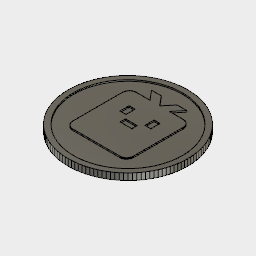
Tomato Coaster (Autodesk Fusion 360 design; units mm, degrees)
Autodesk Fusion 360 part; units mm, degrees
sketch "tomato" plane through (0, 0, 0) normal (0, 0, 1) x (1, 0, 0)
  line L0 (18.3031, 41.1095) -> (16.1266, 42.0111)
  line L1 (-21.8898, 21.7819) -> (-21.7279, 21.9929)
  line L2 (-22.0404, 21.5628) -> (-21.8898, 21.7819)
  line L3 (40.0953, 20.4296) -> (38.9711, 22.5)
  line L4 (22.853, 19.0619) -> (22.86, 18.796)
  line L5 (38.9711, 22.5) -> (37.7402, 24.5087)
  line L6 (-18.5747, 23.8134) -> (-18.311, 23.8482)
  line L7 (-30.1109, -33.4415) -> (-28.3194, -34.9716)
  line L8 (7.112, 12.4968) -> (7.112, 5.588)
  line L9 (-4.4196, 2.54) -> (-4.4196, -1.524)
  line L10 (-26.4503, -36.4058) -> (-24.5087, -37.7402)
  line L11 (44.7535, -4.7038) -> (44.9383, -2.3551)
  line L12 (28.3194, 34.9716) -> (26.4503, 36.4058)
  line L13 (-21.5552, 22.1952) -> (-21.3721, 22.3881)
  line L14 (42.0111, -16.1266) -> (42.7975, -13.9058)
  line L15 (-19.6005, 23.5386) -> (-19.3498, 23.6273)
  line L16 (-22.4208, -20.8622) -> (-22.5226, -20.6165)
  line L17 (-19.3498, 23.6273) -> (-19.0948, 23.7029)
  line L18 (-21.7279, 21.9929) -> (-21.5552, 22.1952)
  line L19 (20.0863, -23.3223) -> (19.8462, -23.4368)
  line L20 (-22.853, 19.0619) -> (-22.8322, 19.327)
  line L21 (-22.8322, 19.327) -> (-22.7975, 19.5907)
  line L22 (-30.1109, 33.4415) -> (-31.8198, 31.8198)
  line L23 (20.32, -23.1954) -> (20.0863, -23.3223)
  line L24 (19.8462, -23.4368) -> (19.6005, -23.5386)
  line L25 (19.6005, -23.5386) -> (19.3498, -23.6273)
  line L26 (11.5824, 12.4968) -> (7.112, 12.4968)
  line L27 (17.78, -23.876) -> (-17.78, -23.876)
  line L28 (22.5, 38.9711) -> (20.4296, 40.0953)
  line L29 (-34.9716, 28.3194) -> (-36.4058, 26.4503)
  line L30 (33.4415, -30.1109) -> (34.9716, -28.3194)
  line L31 (7.112, 5.588) -> (11.5824, 5.588)
  line L32 (44.446, -7.0396) -> (44.7535, -4.7038)
  line L33 (20.9769, -22.7439) -> (20.7659, -22.9058)
  line L34 (22.5, -38.9711) -> (24.5087, -37.7402)
  line L35 (-21.1792, -22.5712) -> (-21.3721, -22.3881)
  line L36 (-20.9769, -22.7439) -> (-21.1792, -22.5712)
  line L37 (19.0948, 23.7029) -> (19.3498, 23.6273)
  line L38 (-37.7402, -24.5087) -> (-36.4058, -26.4503)
  line L39 (31.8198, -31.8198) -> (33.4415, -30.1109)
  line L40 (36.4058, -26.4503) -> (37.7402, -24.5087)
  line L41 (-20.9769, 22.7439) -> (-20.7659, 22.9058)
  line L42 (37.7402, -24.5087) -> (38.9711, -22.5)
  line L43 (-20.32, 23.1954) -> (-20.0863, 23.3223)
  line L44 (-20.0863, 23.3223) -> (-19.8462, 23.4368)
  line L45 (-24.5087, -37.7402) -> (-22.5, -38.9711)
  line L46 (-21.1792, 22.5712) -> (-20.9769, 22.7439)
  line L47 (-20.5468, 23.0564) -> (-20.32, 23.1954)
  line L48 (-20.7659, 22.9058) -> (-20.5468, 23.0564)
  line L49 (-21.3721, 22.3881) -> (-21.1792, 22.5712)
  line L50 (44.0166, -9.356) -> (44.446, -7.0396)
  line L51 (-11.6469, -43.4667) -> (-9.356, -44.0166)
  line L52 (-13.9058, -42.7975) -> (-11.6469, -43.4667)
  line L53 (-16.1266, -42.0111) -> (-13.9058, -42.7975)
  line L54 (-18.3031, -41.1095) -> (-16.1266, -42.0111)
  line L55 (-20.4296, -40.0953) -> (-18.3031, -41.1095)
  line L56 (22.1794, 21.336) -> (22.3063, 21.1023)
  line L57 (19.3498, 23.6273) -> (19.6005, 23.5386)
  line L58 (20.32, 23.1954) -> (20.5468, 23.0564)
  line L59 (20.0863, 23.3223) -> (20.32, 23.1954)
  line L60 (-11.5824, 5.588) -> (-7.112, 5.588)
  line L61 (43.4667, -11.6469) -> (44.0166, -9.356)
  line L62 (9.356, 44.0166) -> (7.0396, 44.446)
  line L63 (13.9058, -42.7975) -> (16.1266, -42.0111)
  line L64 (26.4503, 36.4058) -> (24.5087, 37.7402)
  line L65 (5.9677, 30.988) -> (13.2829, 30.988)
  line L66 (13.2829, 30.988) -> (7.3152, 23.876)
  line L67 (-13.9058, 42.7975) -> (-16.1266, 42.0111)
  line L68 (24.5087, 37.7402) -> (22.5, 38.9711)
  line L69 (-11.6469, 43.4667) -> (-13.9058, 42.7975)
  line L70 (13.9058, 42.7975) -> (11.6469, 43.4667)
  line L71 (-20.4296, 40.0953) -> (-22.5, 38.9711)
  line L72 (22.0404, -21.5628) -> (21.8898, -21.7819)
  line L73 (-45, 0) -> (-44.9383, -2.3551)
  line L74 (-44.9383, 2.3551) -> (-45, 0)
  line L75 (-18.3031, 41.1095) -> (-20.4296, 40.0953)
  line L76 (-43.4667, -11.6469) -> (-42.7975, -13.9058)
  line L77 (22.7975, 19.5907) -> (22.8322, 19.327)
  line L78 (22.6114, 20.3658) -> (22.6869, 20.1108)
  line L79 (22.6869, 20.1108) -> (22.749, 19.8522)
  line L80 (22.749, 19.8522) -> (22.7975, 19.5907)
  line L81 (22.5226, 20.6165) -> (22.6114, 20.3658)
  line L82 (-44.7535, 4.7038) -> (-44.9383, 2.3551)
  line L83 (-28.3194, -34.9716) -> (-26.4503, -36.4058)
  line L84 (-44.9383, -2.3551) -> (-44.7535, -4.7038)
  line L85 (-31.8198, -31.8198) -> (-30.1109, -33.4415)
  line L86 (-42.7975, -13.9058) -> (-42.0111, -16.1266)
  line L87 (-41.1095, -18.3031) -> (-40.0953, -20.4296)
  line L88 (-42.0111, -16.1266) -> (-41.1095, -18.3031)
  line L89 (26.4503, -36.4058) -> (28.3194, -34.9716)
  line L90 (24.5087, -37.7402) -> (26.4503, -36.4058)
  line L91 (34.9716, -28.3194) -> (36.4058, -26.4503)
  line L92 (-2.3551, 44.9383) -> (-4.7038, 44.7535)
  line L93 (-9.356, -44.0166) -> (-7.0396, -44.446)
  line L94 (-5.9677, 30.988) -> (0, 23.876)
  line L95 (-44.0166, -9.356) -> (-43.4667, -11.6469)
  line L96 (-4.7038, 44.7535) -> (-7.0396, 44.446)
  line L97 (-22.1794, -21.336) -> (-22.3063, -21.1023)
  line L98 (22.6869, -20.1108) -> (22.6114, -20.3658)
  line L99 (18.5747, -23.8134) -> (18.311, -23.8482)
  line L100 (22.5226, -20.6165) -> (22.4208, -20.8622)
  line L101 (22.6114, -20.3658) -> (22.5226, -20.6165)
  line L102 (22.749, -19.8522) -> (22.6869, -20.1108)
  line L103 (22.86, 18.796) -> (22.86, -18.796)
  line L104 (22.3063, 21.1023) -> (22.4208, 20.8622)
  line L105 (-36.4058, -26.4503) -> (-34.9716, -28.3194)
  line L106 (22.4208, 20.8622) -> (22.5226, 20.6165)
  line L107 (22.4208, -20.8622) -> (22.3063, -21.1023)
  line L108 (22.853, -19.0619) -> (22.8322, -19.327)
  line L109 (22.86, -18.796) -> (22.853, -19.0619)
  line L110 (22.8322, -19.327) -> (22.7975, -19.5907)
  line L111 (-34.9716, -28.3194) -> (-33.4415, -30.1109)
  line L112 (20.9769, 22.7439) -> (21.1792, 22.5712)
  line L113 (4.4196, 2.54) -> (-4.4196, 2.54)
  line L114 (-22.5, -38.9711) -> (-20.4296, -40.0953)
  line L115 (-20.0863, -23.3223) -> (-20.32, -23.1954)
  line L116 (-19.8462, -23.4368) -> (-20.0863, -23.3223)
  line L117 (-19.3498, -23.6273) -> (-19.6005, -23.5386)
  line L118 (-19.6005, -23.5386) -> (-19.8462, -23.4368)
  line L119 (-7.112, 5.588) -> (-7.112, 12.4968)
  line L120 (-4.4196, -1.524) -> (4.4196, -1.524)
  line L121 (18.311, -23.8482) -> (18.0459, -23.869)
  line L122 (40.0953, -20.4296) -> (41.1095, -18.3031)
  line L123 (20.7659, -22.9058) -> (20.5468, -23.0564)
  line L124 (38.9711, -22.5) -> (40.0953, -20.4296)
  line L125 (30.1109, -33.4415) -> (31.8198, -31.8198)
  line L126 (28.3194, -34.9716) -> (30.1109, -33.4415)
  line L127 (-22.8322, -19.327) -> (-22.853, -19.0619)
  line L128 (19.0948, -23.7029) -> (18.8362, -23.765)
  line L129 (18.8362, -23.765) -> (18.5747, -23.8134)
  line L130 (18.0459, -23.869) -> (17.78, -23.876)
  line L131 (-7.3152, 23.876) -> (-13.2829, 30.988)
  line L132 (2.3551, -44.9383) -> (4.7038, -44.7535)
  line L133 (4.7038, -44.7535) -> (7.0396, -44.446)
  line L134 (21.1792, -22.5712) -> (20.9769, -22.7439)
  line L135 (22.7975, -19.5907) -> (22.749, -19.8522)
  line L136 (-40.0953, -20.4296) -> (-38.9711, -22.5)
  line L137 (-37.7402, 24.5087) -> (-38.9711, 22.5)
  line L138 (-44.7535, -4.7038) -> (-44.446, -7.0396)
  line L139 (11.5824, 5.588) -> (11.5824, 12.4968)
  line L140 (19.3498, -23.6273) -> (19.0948, -23.7029)
  line L141 (16.1266, 42.0111) -> (13.9058, 42.7975)
  line L142 (7.0396, -44.446) -> (9.356, -44.0166)
  line L143 (-22.0404, -21.5628) -> (-22.1794, -21.336)
  line L144 (-31.8198, 31.8198) -> (-33.4415, 30.1109)
  line L145 (-33.4415, 30.1109) -> (-34.9716, 28.3194)
  line L146 (-33.4415, -30.1109) -> (-31.8198, -31.8198)
  line L147 (-36.4058, 26.4503) -> (-37.7402, 24.5087)
  line L148 (4.7038, 44.7535) -> (2.3551, 44.9383)
  line L149 (9.356, -44.0166) -> (11.6469, -43.4667)
  line L150 (22.1794, -21.336) -> (22.0404, -21.5628)
  line L151 (21.7279, -21.9929) -> (21.5552, -22.1952)
  line L152 (21.8898, -21.7819) -> (21.7279, -21.9929)
  line L153 (21.3721, -22.3881) -> (21.1792, -22.5712)
  line L154 (21.5552, -22.1952) -> (21.3721, -22.3881)
  line L155 (4.4196, -1.524) -> (4.4196, 2.54)
  line L156 (22.8322, 19.327) -> (22.853, 19.0619)
  line L157 (22.3063, -21.1023) -> (22.1794, -21.336)
  line L158 (33.4415, 30.1109) -> (31.8198, 31.8198)
  line L159 (44.7535, 4.7038) -> (44.446, 7.0396)
  line L160 (44.9383, 2.3551) -> (44.7535, 4.7038)
  line L161 (34.9716, 28.3194) -> (33.4415, 30.1109)
  line L162 (42.7975, 13.9058) -> (42.0111, 16.1266)
  line L163 (43.4667, 11.6469) -> (42.7975, 13.9058)
  line L164 (16.1266, -42.0111) -> (18.3031, -41.1095)
  line L165 (-22.86, -18.796) -> (-22.86, 18.796)
  line L166 (-18.0459, -23.869) -> (-18.311, -23.8482)
  line L167 (-22.749, 19.8522) -> (-22.6869, 20.1108)
  line L168 (-2.3551, -44.9383) -> (0, -45)
  line L169 (-22.7975, 19.5907) -> (-22.749, 19.8522)
  line L170 (-22.86, 18.796) -> (-22.853, 19.0619)
  line L171 (-7.0396, -44.446) -> (-4.7038, -44.7535)
  line L172 (-4.7038, -44.7535) -> (-2.3551, -44.9383)
  line L173 (-42.0111, 16.1266) -> (-42.7975, 13.9058)
  line L174 (-17.78, -23.876) -> (-18.0459, -23.869)
  line L175 (-22.749, -19.8522) -> (-22.7975, -19.5907)
  line L176 (-22.7975, -19.5907) -> (-22.8322, -19.327)
  line L177 (0, -45) -> (2.3551, -44.9383)
  line L178 (-22.6114, -20.3658) -> (-22.6869, -20.1108)
  line L179 (-18.311, -23.8482) -> (-18.5747, -23.8134)
  line L180 (-22.4208, 20.8622) -> (-22.3063, 21.1023)
  line L181 (-22.5226, 20.6165) -> (-22.4208, 20.8622)
  line L182 (-19.0948, -23.7029) -> (-19.3498, -23.6273)
  line L183 (-18.8362, -23.765) -> (-19.0948, -23.7029)
  line L184 (-22.6114, 20.3658) -> (-22.5226, 20.6165)
  line L185 (-22.6869, 20.1108) -> (-22.6114, 20.3658)
  line L186 (-19.8462, 23.4368) -> (-19.6005, 23.5386)
  line L187 (-18.5747, -23.8134) -> (-18.8362, -23.765)
  line L188 (-22.1794, 21.336) -> (-22.0404, 21.5628)
  line L189 (-22.3063, 21.1023) -> (-22.1794, 21.336)
  line L190 (-22.6869, -20.1108) -> (-22.749, -19.8522)
  line L191 (-41.1095, 18.3031) -> (-42.0111, 16.1266)
  line L192 (-42.7975, 13.9058) -> (-43.4667, 11.6469)
  line L193 (-43.4667, 11.6469) -> (-44.0166, 9.356)
  line L194 (21.7279, 21.9929) -> (21.8898, 21.7819)
  line L195 (-44.0166, 9.356) -> (-44.446, 7.0396)
  line L196 (-44.446, 7.0396) -> (-44.7535, 4.7038)
  line L197 (-38.9711, 22.5) -> (-40.0953, 20.4296)
  line L198 (-40.0953, 20.4296) -> (-41.1095, 18.3031)
  line L199 (22.0404, 21.5628) -> (22.1794, 21.336)
  line L200 (21.8898, 21.7819) -> (22.0404, 21.5628)
  line L201 (20.5468, -23.0564) -> (20.32, -23.1954)
  line L202 (-9.356, 44.0166) -> (-11.6469, 43.4667)
  line L203 (-20.32, -23.1954) -> (-20.5468, -23.0564)
  line L204 (20.4296, 40.0953) -> (18.3031, 41.1095)
  line L205 (-20.7659, -22.9058) -> (-20.9769, -22.7439)
  line L206 (19.8462, 23.4368) -> (20.0863, 23.3223)
  line L207 (7.3152, 23.876) -> (17.78, 23.876)
  line L208 (21.1792, 22.5712) -> (21.3721, 22.3881)
  line L209 (21.3721, 22.3881) -> (21.5552, 22.1952)
  line L210 (21.5552, 22.1952) -> (21.7279, 21.9929)
  line L211 (19.6005, 23.5386) -> (19.8462, 23.4368)
  line L212 (-21.3721, -22.3881) -> (-21.5552, -22.1952)
  line L213 (7.0396, 44.446) -> (4.7038, 44.7535)
  line L214 (20.4296, -40.0953) -> (22.5, -38.9711)
  line L215 (-20.5468, -23.0564) -> (-20.7659, -22.9058)
  line L216 (20.5468, 23.0564) -> (20.7659, 22.9058)
  line L217 (-21.5552, -22.1952) -> (-21.7279, -21.9929)
  line L218 (11.6469, -43.4667) -> (13.9058, -42.7975)
  line L219 (20.7659, 22.9058) -> (20.9769, 22.7439)
  line L220 (18.5747, 23.8134) -> (18.8362, 23.765)
  line L221 (-7.112, 12.4968) -> (-11.5824, 12.4968)
  line L222 (-11.5824, 12.4968) -> (-11.5824, 5.588)
  line L223 (-26.4503, 36.4058) -> (-28.3194, 34.9716)
  line L224 (-28.3194, 34.9716) -> (-30.1109, 33.4415)
  line L225 (-24.5087, 37.7402) -> (-26.4503, 36.4058)
  line L226 (-22.5, 38.9711) -> (-24.5087, 37.7402)
  line L227 (-22.3063, -21.1023) -> (-22.4208, -20.8622)
  line L228 (-44.446, -7.0396) -> (-44.0166, -9.356)
  line L229 (-19.0948, 23.7029) -> (-18.8362, 23.765)
  line L230 (0, 23.876) -> (5.9677, 30.988)
  line L231 (-17.78, 23.876) -> (-7.3152, 23.876)
  line L232 (-18.311, 23.8482) -> (-18.0459, 23.869)
  line L233 (-21.7279, -21.9929) -> (-21.8898, -21.7819)
  line L234 (18.8362, 23.765) -> (19.0948, 23.7029)
  line L235 (11.6469, 43.4667) -> (9.356, 44.0166)
  line L236 (-16.1266, 42.0111) -> (-18.3031, 41.1095)
  line L237 (2.3551, 44.9383) -> (0, 45)
  line L238 (45, 0) -> (44.9383, 2.3551)
  line L239 (44.9383, -2.3551) -> (45, 0)
  line L240 (-18.8362, 23.765) -> (-18.5747, 23.8134)
  line L241 (44.446, 7.0396) -> (44.0166, 9.356)
  line L242 (41.1095, 18.3031) -> (40.0953, 20.4296)
  line L243 (42.0111, 16.1266) -> (41.1095, 18.3031)
  line L244 (36.4058, 26.4503) -> (34.9716, 28.3194)
  line L245 (37.7402, 24.5087) -> (36.4058, 26.4503)
  line L246 (-13.2829, 30.988) -> (-5.9677, 30.988)
  line L247 (31.8198, 31.8198) -> (30.1109, 33.4415)
  line L248 (30.1109, 33.4415) -> (28.3194, 34.9716)
  line L249 (44.0166, 9.356) -> (43.4667, 11.6469)
  line L250 (17.78, 23.876) -> (18.0459, 23.869)
  line L251 (18.0459, 23.869) -> (18.311, 23.8482)
  line L252 (-18.0459, 23.869) -> (-17.78, 23.876)
  line L253 (-38.9711, -22.5) -> (-37.7402, -24.5087)
  line L254 (-22.5226, -20.6165) -> (-22.6114, -20.3658)
  line L255 (18.311, 23.8482) -> (18.5747, 23.8134)
  line L256 (-7.0396, 44.446) -> (-9.356, 44.0166)
  line L257 (-21.8898, -21.7819) -> (-22.0404, -21.5628)
  line L258 (0, 45) -> (-2.3551, 44.9383)
  line L259 (-22.853, -19.0619) -> (-22.86, -18.796)
  line L260 (18.3031, -41.1095) -> (20.4296, -40.0953)
  line L261 (42.7975, -13.9058) -> (43.4667, -11.6469)
  line L262 (41.1095, -18.3031) -> (42.0111, -16.1266)
sketch "Sketch2" plane through (0, 0, 0) normal (0, 0, 1) x (1, 0, 0)
  circle A0 centre (0, 0) radius 41
  constraint coincident A0.centre origin
extrude "Extrude4" add sketch "tomato" along normal blind 5 contours L0 L3 L5 L7 L10 L11 L12 L14 L22 L28 L29 L30 L32 L34 L38 L39 L40 L42 L45 L50 L51 L52 L53 L54 L55 L61 L62 L63 L64 L67 L68 L69 L70 L71 L73 L74 L75 L76 L82 L83 L84 L85 L86 L87 L88 L89 L90 L91 L92 L93 L95 L96 L105 L111 L114 L122 L124 L125 L126 L132 L133 L136 L137 L138 L141 L142 L144 L145 L146 L147 L148 L149 L158 L159 L160 L161 L162 L163 L164 L168 L171 L172 L173 L177 L191 L192 L193 L195 L196 L197 L198 L202 L204 L213 L214 L218 L223 L224 L225 L226 L228 L235 L236 L237 L238 L239 L241 L242 L243 L244 L245 L247 L248 L249 L253 L256 L258 L260 L261 L262
extrude "Extrude5" cut sketch "Sketch2" along normal blind 5
extrude "Extrude6" add sketch "Sketch2" along normal blind 4
extrude "Extrude7" add sketch "tomato" along normal blind 1 from surface at 4 contours L1 L2 L4 L6 L13 L15 L16 L17 L18 L19 L20 L21 L23 L24 L25 L27 L33 L35 L36 L37 L41 L43 L44 L46 L47 L48 L49 L56 L57 L58 L59 L65 L66 L72 L77 L78 L79 L80 L81 L94 L97 L98 L99 L100 L101 L102 L103 L104 L106 L107 L108 L109 L110 L112 L115 L116 L117 L118 L121 L123 L127 L128 L129 L130 L131 L134 L135 L140 L143 L150 L151 L152 L153 L154 L156 L157 L165 L166 L167 L169 L170 L174 L175 L176 L178 L179 L180 L181 L182 L183 L184 L185 L186 L187 L188 L189 L190 L194 L199 L200 L201 L203 L205 L206 L207 L208 L209 L210 L211 L212 L215 L216 L217 L219 L220 L227 L229 L230 L231 L232 L233 L234 L240 L246 L250 L251 L252 L254 L255 L257 L259
extrude "Extrude2" [suppressed]
extrude "Extrude3" [suppressed]
extrude "Extrude1" [suppressed]
